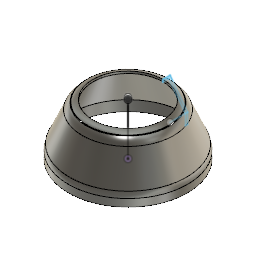
case (Autodesk Fusion 360 design; units mm, degrees)
Autodesk Fusion 360 part; units mm, degrees
sketch "Sketch1" plane through (0, 0, 0) normal (1, 0, 0) x (0, 1, 0)
  line L0 (0, 76) -> (0, 73)
  line L1 (85, 0) -> (85, 15)
  line L2 (85, 0) -> (82, 0)
  line L3 (82, 0) -> (82, 15)
  line L4 (0, 0) -> (0, 73)
  line L5 (85, 15) -> (60, 15)
  line L6 (60, 73) -> (85, 15)
  line L7 (60, 73) -> (50, 73)
  line L8 (50, 73) -> (50, 70)
  line L9 (50, 70) -> (58.2931, 70)
  line L10 (58.2931, 70) -> (82, 15)
  dimension "d21" = 3
  dimension "d23" = 15
  dimension "d24" = 85
  dimension "d38" = 73
  dimension "d39" = 25
  dimension "d40" = 10
  dimension "d41" = 3
  constraint perpendicular L2 L3
  constraint coincident L4.start origin
  constraint vertical L4
  constraint perpendicular L3 L5
  constraint perpendicular L7 L8
  constraint parallel L6 L10
  measures "d21" distance of L1.start L2.end
  measures "d23" distance of L2.end L3.end
  measures "d24" distance of L4.start L1.start
  measures "d38" distance of L4.start L0.end
  measures "d39" distance of L1.end L5.end
  measures "d40" distance of L7.end L6.start
  measures "d41" distance of L7.end L8.end
revolve "Revolve1" add sketch "Sketch1" angle 360 about axis through (0, 0, 1.75) along (0, 0, 1)
fillet "Fillet1" [no effect]
sketch "Sketch2" plane through (0, 0, 0) normal (0, 0, 1) x (1, 0, 0)
fillet "Fillet2" radius 20 1 faces at (-73.9527, -29.0243, 27.8889)
